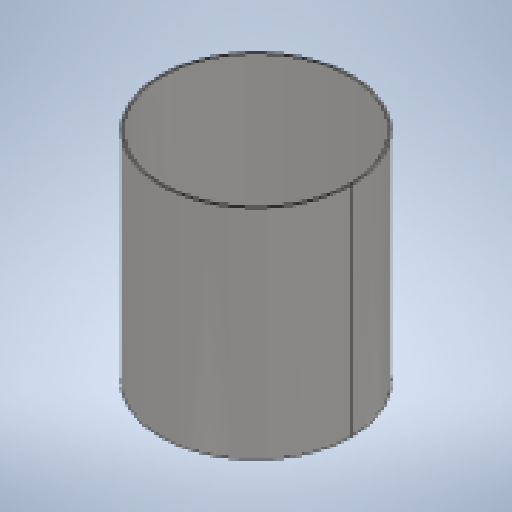
# Autodesk Inventor part: TKS 3103 TOP DS outer tube
Saved by Autodesk Inventor 2025.3 (Build 293356030, 356C)
## iProperties
Created: 2025-02-19
Part Number: TKS 3103 TOP DS outer tube
Material: Stainless Steel
Document SubType Name: Sheet Metal
Designer: user
Density: 8 g/cm^3
Appearance: Semi-Polished
Flat Pattern Width: 24 cm
Flat Pattern Length: 65.2516 cm
Flat Pattern Area: 1566.04 cm^2
Sheet Metal Rule: Default
Sheet Metal Width: 240,000 mm
Sheet Metal Length: 652,516 mm
Sheet Metal Area: 156603,836 mm^2
Author: admin
Autodesk Inventor part; units mm, degrees
ref_plane "YZ Plane" through (0, 0, 0) normal (1, 0, 0) x (0, 1, 0)
ref_plane "XZ Plane" through (0, 0, 0) normal (0, 1, 0) x (-1, 0, 0)
ref_plane "XY Plane" through (0, 0, 0) normal (0, 0, 1) x (1, 0, 0)
sketch "Sketch2" plane through (0, 0, 0) normal (0, 1, 0) x (-1, 0, 0)
  line L0 (0, 0) -> (0, 275.0943)
  line L1 (-103, 30) -> (-105, 30)
  line L2 (-105, 30) -> (-105, 270)
  line L3 (-105, 270) -> (-103, 270)
  line L4 (-103, 270) -> (-103, 30)
  dimension "d4" = 240
  dimension "d5" = 2
  dimension "d6" = 210
  constraints: 10 end point, 2 parallel, 1 horizontal, 1 perpendicular, 1 vertical
  measures "d4" distance of L1.end L2.end
  measures "d5" distance of L2.end L3.end
  measures "d6" diameter of L2 L0
revolve "Revolution1" add sketch "Sketch2" angle 359.9 about axis through (0, 0, 0) along (0, 0, 1)
equation "\"d5\" = Thickness"
equation "\"BendRadius\" = Thickness"
equation "\"BendReliefWidth\" = Thickness"
equation "\"BendReliefDepth\" = 0.5 * Thickness"
equation "\"CornerReliefSize\" = 4 * Thickness"
equation "\"MinimumRemnant\" = 2 * Thickness"
equation "\"TransitionRadius\" = BendRadius"
equation "\"JacobiRadiusSize\" = BendRadius"
equation "\"GapSize\" = Thickness"
equation "\"Thickness\" = 2"
body "Solid2"
